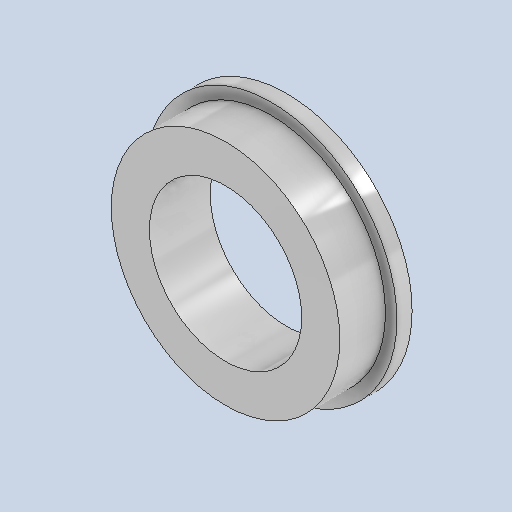
# Autodesk Inventor part: bear_10_15_sn_CPY_CPY
Saved by Autodesk Inventor 2024.1 (Build 281209000, 209)
## iProperties
Created: 2021-04-20
Part Number: bear_10_15_sn_CPY_CPY
Material: アルミニウム 6061-AHC
Document SubType Name: Modeling
Designer: haruy
Density: 2.7 g/cm^3
Appearance: アルミニウム - ダーク
Author: 中島 青蔵
Autodesk Inventor part; units mm, degrees
ref_plane "YZ Plane" through (0, 0, 0) normal (1, 0, 0) x (0, 1, 0)
ref_plane "XZ Plane" through (0, 0, 0) normal (0, 1, 0) x (-1, 0, 0)
ref_plane "XY Plane" through (0, 0, 0) normal (0, 0, 1) x (1, 0, 0)
sketch "スケッチ1" plane through (0, 0, 0) normal (0, 0, 1) x (1, 0, 0)
  circle A0 centre (0, 0) radius 5
  circle A1 centre (0, 0) radius 7.5
  circle A2 centre (0, 0) radius 8.25
  dimension "d0" = 10
  dimension "d1" = 15
  dimension "d2" = 16.5
  constraints: 3 centre point, 3 coincident
  measures "d0" diameter of A0
  measures "d1" diameter of A1
  measures "d2" diameter of A2
extrude "押し出し1" add sketch "スケッチ1" along normal blind 1 contours A2
extrude "押し出し2" add sketch "スケッチ1" along normal blind 4 contours A1
